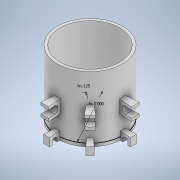
# Autodesk Inventor part: roundMouseSupport
Saved by Autodesk Inventor 2022 (Build 260153000, 153)
## iProperties
Created: 2021-04-17
Part Number: roundMouseSupport
Material: Generic
Document SubType Name: Modeling
Designer: robst
Density: 1 g/cm^3
Appearance: Default
Author: robst
Autodesk Inventor part; units mm, degrees
ref_plane "YZ Plane" through (0, 0, 0) normal (1, 0, 0) x (0, 1, 0)
ref_plane "XZ Plane" through (0, 0, 0) normal (0, 1, 0) x (-1, 0, 0)
ref_plane "XY Plane" through (0, 0, 0) normal (0, 0, 1) x (1, 0, 0)
sketch "Sketch8" plane through (0, 0, 0) normal (0, 1, 0) x (-1, 0, 0)
  circle A0 centre (0, 0) radius 38.1
  circle A1 centre (0, 0) radius 34.925
  dimension "d25" = 76.2
  dimension "d26" = 3.175
  constraints: 2 centre point, 2 coincident
  measures "d25" diameter of A0
  measures "d26" radial gap between concentric circles of A1 A0
extrude "Extrusion6" add sketch "Sketch8" against normal blind 3.81 contours A0 | A1
extrude "Extrusion7" add sketch "Sketch8" along normal blind 72.39
sketch "Sketch9" plane through (0, -3.81, 0) normal (0, -1, 0) x (1, 0, 0)
  point P0 (0, 0)
sketch "Sketch10" plane through (0, 0, 0) normal (1, 0, 0) x (0, 1, 0)
  line L0 (72.39, 38.1) -> (-3.81, 38.1) projected
  line L1 (-3.81, 38.1) -> (-3.81, 50.8)
  line L2 (-3.81, 50.8) -> (5.715, 50.8)
  line L3 (5.715, 50.8) -> (5.715, 38.1)
  arc A0 (-0.635, 41.275) -> (-0.635, 47.625) centre (-0.635, 44.45) ccw
  line L4 (-3.81, 38.1) -> (-3.81, -38.1) projected
  line L5 (-0.635, 47.625) -> (-3.81, 47.625)
  line L6 (-0.635, 41.275) -> (-3.81, 41.275)
  line L7 (-16.51, 0) -> (72.39, 0) projected
  point P0 (0, 0)
  dimension "d31" = 6.35
  dimension "d32" = 3.175
  dimension "d35" = 3.175
  dimension "d36" = 3.175
  constraints: 10 end point, 4 perpendicular, 4 point on line, 3 tangent, 2 point on circle, 1 centre point, 1 collinear, 1 vertical
  measures "d31" diameter of A0
  measures "d32" distance edge to line of A0 L2
  measures "d35" distance edge to line of A0 L0
  measures "d36" distance edge to line of A0 L3
revolve "Revolution1" add sketch "Sketch10" angle 8 mid plane about axis through (0, -10, 0) along (0, 1, 0) contours L0 L1 L6 A0 L5 L2 L3
sketch "Sketch11" plane through (0, 0, 0) normal (1, 0, 0) x (0, 1, 0)
  line L0 (72.39, 38.1) -> (5.715, 38.1) projected
  arc A0 (26.8199, 45.5701) -> (35.4101, 45.5701) centre (31.115, 45.5701) ccw
  line L1 (38.5851, 38.1) -> (38.5851, 53.0402)
  line L2 (23.6449, 53.0402) -> (23.6449, 38.1)
  line L3 (35.4101, 45.5701) -> (35.4101, 53.0402)
  line L4 (26.8199, 45.5701) -> (26.8199, 53.0402)
  line L5 (38.5851, 53.0402) -> (35.4101, 53.0402)
  line L6 (26.8199, 53.0402) -> (23.6449, 53.0402)
  line L7 (-16.51, 0) -> (72.39, 0) projected
  arc A1 (2.54, 44.45) -> (-0.635, 47.625) centre (-0.635, 44.45) ccw projected
  arc A2 (-0.635, 41.275) -> (2.54, 44.45) centre (-0.635, 44.45) ccw projected
  point P0 (0, 0)
  dimension "d38" = 8.5902
  dimension "d39" = 3.175
  dimension "d40" = 3.175
  dimension "d41" = 3.175
  dimension "d44" = 31.75
  constraints: 12 end point, 8 perpendicular, 2 point on circle, 2 point on line, 2 tangent, 1 centre point
  measures "d38" diameter of A0
  measures "d39" distance edge to line of A0 L0
  measures "d40" distance edge to line of A0 L1
  measures "d41" distance edge to line of A0 L2
  measures "d44" horizontal distance of A0.centre A1.centre
revolve "Revolution2" add sketch "Sketch11" angle 10 mid plane about axis through (0, -10, 0) along (0, 1, 0)
pattern_circular "Circular Pattern2" count 3 over 90 about axis through (0, -10, 0) along (0, 1, 0) of "Revolution2", "Revolution1"
equation "\"d25\" = outerDiameter"
equation "\"d26\" = wallThickness"
equation "\"d27\" = floorThickness"
equation "\"d29\" = height - floorThickness"
equation "\"d31\" = holeDiameter"
equation "\"d32\" = fromWallToHole"
equation "\"d35\" = fromEdgeToWall"
equation "\"d36\" = htAboveHole"
equation "\"d39\" = fromWallToHole"
equation "\"d40\" = htAboveHole"
equation "\"d41\" = htAboveHole"
equation "\"d44\" = spaceBetweenWire"
equation "\"htAboveHole\" = 3.175"
equation "\"fromWallToHole\" = 3.175"
equation "\"fromEdgeToWall\" = 3.175"
equation "\"holeDiameter\" = 6.35"
equation "\"bottomHeight\" = holeDiameter + htAboveHole"
equation "\"d42\" = fromEdgeToWall"
equation "\"outerDiameter\" = 76.2"
equation "\"floorThickness\" = 3.81"
equation "\"wallThickness\" = 3.175"
equation "\"spaceBetweenWire\" = 31.75"
equation "\"height\" = 76.2"
body "Solid2"
